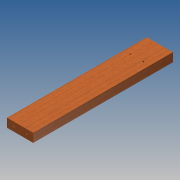
# Autodesk Inventor part: 2p2psh1
Saved by Autodesk Inventor 2014 SP1 (Build 180222100, 222)
## iProperties
Company: HERA Project
Created: 2013-09-03
Part Number: 2p2psh1
Material: Wood (Cherry)
Document SubType Name: Modeling
Designer: David DeBoer
Mass: 1030.35 g
Surface Area: 1640.3 cm^2
Volume: 2060.71 cm^3
Density: 0.5 g/cm^3
Description: pole stand support horizontal 1
Appearance: Cherry - Natural Low Gloss
Author: David DeBoer
Autodesk Inventor part; units mm, degrees
ref_plane "YZ Plane" through (0, 0, 0) normal (1, 0, 0) x (0, 1, 0)
ref_plane "XZ Plane" through (0, 0, 0) normal (0, 1, 0) x (-1, 0, 0)
ref_plane "XY Plane" through (0, 0, 0) normal (0, 0, 1) x (1, 0, 0)
sketch "Sketch1" plane through (0, 0, 0) normal (0, 0, 1) x (1, 0, 0)
  line L0 (0, 0) -> (114, 0)
  line L1 (114, 0) -> (114, 38)
  line L2 (114, 38) -> (0, 38)
  line L3 (0, 38) -> (0, 0)
  dimension "d0" = 114
  dimension "d1" = 38
  constraints: 8 end point, 2 parallel, 1 horizontal, 1 perpendicular
  measures "d0" distance of L0.start L0.end
  measures "d1" distance of L2.end L0.start
extrude "Extrusion1" add sketch "Sketch1" along normal blind 609.6
sketch "Sketch2" plane through (0, 0, 609.6) normal (0, 0, 1) x (1, 0, 0)
  line L0 (0, 0) -> (114, 0) projected
  circle A0 centre (28.5, 19) radius 5.7238
  circle A1 centre (85.5, 19) radius 5.7238
  line L1 (114, 38) -> (0, 38) projected
  line L2 (57, 38) -> (57, 0) construction
  line L3 (28.5, 19) -> (85.5, 19) construction
  line L4 (57, 19) -> (57, 23.2884) construction
  dimension "d7" = 57
  constraints: 6 end point, 4 midpoint, 2 centre point, 2 perpendicular, 1 horizontal, 2 other
  measures "d7" distance of L3.start L3.end
hole "Hole1" at (28.5, 19, 609.6) at (85.5, 19, 609.6) direction (0, 0, -1) diameter 6.35 depth 25.4 tip angle 118
sketch "Sketch3" plane through (0, 38, 0) normal (0, 1, 0) x (1, 0, 0)
  line L0 (114, 0) -> (0, 0) projected
  circle A0 centre (28.5, -100) radius 3.5498
  circle A1 centre (85.5, -100) radius 3.5498
  line L1 (114, 0) -> (114, -609.6) projected
  line L2 (57, 0) -> (57, -100) construction
  line L3 (28.5, -100) -> (85.5, -100) construction
  dimension "d23" = 57
  dimension "d36" = 100
  constraints: 4 end point, 2 centre point, 2 midpoint, 1 horizontal, 1 parallel, 1 perpendicular, 2 other
  measures "d23" distance of L3.start L3.end
  measures "d36" distance of L2.end L2.start
hole "Hole2" at (85.5, 38, 100) at (28.5, 38, 100) direction (0, -1, 0) diameter 6.35 end through all
equation "\"d7\" = 0.5 * d0"
equation "\"d23\" = 0.5 * d0"
body "Solid1"
